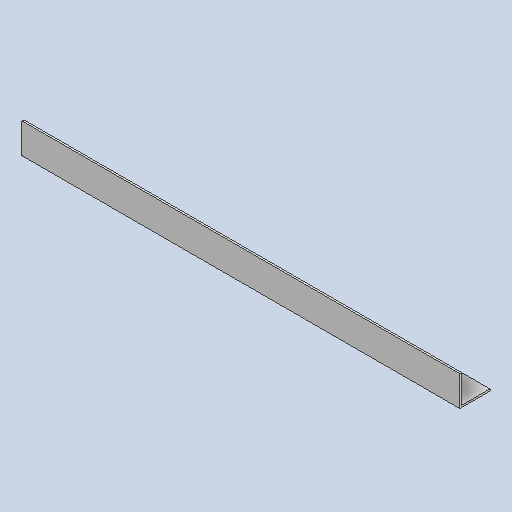
# Autodesk Inventor part: LatL29in
Saved by Autodesk Inventor 2023 (Build 270158030, 158C)
## iProperties
Created: 2022-06-27
Part Number: LatL29in
Material: Generic
Document SubType Name: Modeling
Designer: jeremyy
Density: 1 g/cm^3
Appearance: Default
Author: jeremyy
Autodesk Inventor part; units mm, degrees
ref_plane "YZ Plane" through (0, 0, 0) normal (1, 0, 0) x (0, 1, 0)
ref_plane "XZ Plane" through (0, 0, 0) normal (0, 1, 0) x (-1, 0, 0)
ref_plane "XY Plane" through (0, 0, 0) normal (0, 0, 1) x (1, 0, 0)
sketch "Sketch1" plane through (0, 0, 0) normal (1, 0, 0) x (0, 1, 0)
  line L0 (0, 0) -> (0, -50.8)
  line L1 (0, -50.8) -> (3.175, -50.8)
  line L2 (3.175, -50.8) -> (3.175, -3.175)
  line L3 (3.175, -3.175) -> (50.8, -3.175)
  line L4 (50.8, -3.175) -> (50.8, 0)
  line L5 (50.8, 0) -> (0, 0)
  dimension "d0" = 50.8
  dimension "d1" = 3.175
  dimension "d2" = 47.625
  dimension "d3" = 47.625
  constraints: 12 end point, 4 perpendicular, 1 parallel, 1 vertical
  measures "d0" distance of L0.start L0.end
  measures "d1" distance of L0.end L1.end
  measures "d2" distance of L1.end L2.end
  measures "d3" distance of L2.end L3.end
extrude "Extrusion1" add sketch "Sketch1" along normal blind 736.6
body "Solid1"
